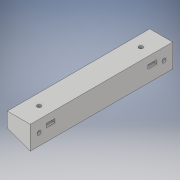
# Autodesk Inventor part: CupHolderBack
Saved by Autodesk Inventor 2019 (Build 230136000, 136)
## iProperties
Created: 2020-12-27
Part Number: CupHolderBack
Material: Типовые
Document SubType Name: Modeling
Designer: Professional
Density: 1 g/cm^3
Appearance: По умолчанию
Author: Professional
Autodesk Inventor part; units mm, degrees
ref_plane "YZ Plane" through (0, 0, 0) normal (1, 0, 0) x (0, 1, 0)
ref_plane "XZ Plane" through (0, 0, 0) normal (0, 1, 0) x (-1, 0, 0)
ref_plane "XY Plane" through (0, 0, 0) normal (0, 0, 1) x (1, 0, 0)
sketch "Эскиз1" plane through (0, 0, 0) normal (0, 0, 1) x (1, 0, 0)
  line L0 (0, 0) -> (0, 10)
  line L1 (0, 10) -> (15.8, 10)
  line L2 (15.8, 10) -> (15.8, -6)
  line L3 (15.8, -6) -> (0, 0)
  dimension "d0" = 10
  dimension "d1" = 15.8
  dimension "d2" = 16
  constraints: 8 end point, 2 perpendicular, 1 vertical
  measures "d0" distance of L0.start L0.end
  measures "d1" distance between parallel lines of L2 L0
  measures "d2" distance of L1.end L2.end
extrude "Выдавливание1" add sketch "Эскиз1" along normal mid plane 98
sketch "Эскиз2" plane through (15.8, -6, 49) normal (1, 0, 0) x (0, 0, -1)
  circle A0 centre (6, 8) radius 1.4
  circle A1 centre (92, 8) radius 1.4
  line L0 (0, 0) -> (98, 0) projected
  line L1 (49, 0) -> (49, 16)
  line L2 (0, 16) -> (98, 16) projected
  point P0 (49, 6)
  dimension "d5" = 8
  dimension "d6" = 86
  dimension "d7" = 2.8
  constraints: 2 centre point, 2 end point, 2 midpoint, 1 other
  measures "d5" distance from line of L2 A0.centre
  measures "d6" distance of A1.centre A0.centre
  measures "d7" diameter of A1
extrude "Выдавливание2" cut sketch "Эскиз2" against normal blind 14
ref_plane "РабПлоскость1" through (0, 5, 49) normal (0, 1, 0) x (1, 0, 0)
sketch "Эскиз4" plane through (0, 5, 49) normal (0, 1, 0) x (1, 0, 0)
  line L0 (15.8, 0) -> (15.8, 98) projected
  line L1 (15.8, 11) -> (4.8, 11)
  line L2 (4.8, 11) -> (4.8, 17)
  line L3 (4.8, 17) -> (15.8, 17)
  line L4 (0, 49) -> (15.8, 49)
  line L5 (15.8, 11) -> (15.8, 17)
  line L6 (15.8, 87) -> (4.8, 87)
  line L7 (4.8, 87) -> (4.8, 81)
  line L8 (4.8, 81) -> (15.8, 81)
  line L9 (15.8, 87) -> (15.8, 81)
  point P0 (15.8, 14)
  point P1 (15.8, 84)
  dimension "d11" = 6
  dimension "d12" = 11
  dimension "d14" = 70
  constraints: 18 end point, 4 symmetric about line, 3 midpoint, 3 perpendicular, 2 horizontal, 2 point on line
  measures "d11" distance of L1.end L2.end
  measures "d12" distance between parallel lines of L0 L2
  measures "d14" distance of point (15.8, 84) point (15.8, 14)
extrude "Выдавливание3" cut sketch "Эскиз4" against normal blind 2.5
sketch "Эскиз5" plane through (0, 10, 49) normal (0, 1, 0) x (1, 0, 0)
  line L0 (15.8, 17) -> (15.8, 11) projected
  line L1 (4.8, 17) -> (15.8, 17) projected
  line L2 (4.8, 11) -> (4.8, 17) projected
  line L3 (15.8, 11) -> (4.8, 11) projected
  line L4 (4.8, 87) -> (15.8, 87) projected
  line L5 (4.8, 81) -> (4.8, 87) projected
  line L6 (15.8, 81) -> (4.8, 81) projected
  line L7 (15.8, 87) -> (15.8, 81) projected
  circle A0 centre (7.9, 14) radius 1.4
  circle A1 centre (7.9, 84) radius 1.4
  line L8 (15.8, 0) -> (0, 0) projected
  point P0 (0, 49)
  point P1 (15.8, 84)
  point P2 (15.8, 14)
  point P3 (7.9, 0)
  dimension "d18" = 2.8
  constraints: 3 midpoint, 2 centre point, 2 horizontal alignment, 2 vertical alignment, 1 equal radius
  measures "d18" diameter of A0
extrude "Выдавливание4" cut sketch "Эскиз5" against normal up to next contours A0 | A1
